Autodesk Fusion 360 part; units mm, degrees
note: some values were not read from the file. Chosen so that the rebuilt part matches the saved one: which face or edge a step refers to; the layout of a text. Set by a fixed rule: which sketch regions a step uses.
(part 2 of 2)
sketch "Sketch18" plane through (0, 0, -22.6) normal (0, 0, -1) x (1, 0, 0)
  line L0 (90.44, 31.25) -> (0.75, 31.25)
  arc A0 (0.75, 31.25) -> (-2.25, 28.25) centre (0.75, 28.25) ccw
  line L1 (-2.25, 28.25) -> (-2.25, 0.75)
  arc A1 (-2.25, 0.75) -> (0.75, -2.25) centre (0.75, 0.75) ccw
  line L2 (0.75, -2.25) -> (90.44, -2.25)
  arc A2 (90.44, -2.25) -> (93.44, 0.75) centre (90.44, 0.75) ccw
  line L3 (93.44, 0.75) -> (93.44, 28.25)
  arc A3 (93.44, 28.25) -> (90.44, 31.25) centre (90.44, 28.25) ccw
  line L4 (2.5, 13.75) -> (2.5, 12)
  line L5 (2.5, 12) -> (1, 12)
  line L6 (1, 12) -> (1, 13.75)
  line L7 (1, 13.75) -> (-0.75, 13.75)
  line L8 (-0.75, 13.75) -> (-0.75, 15.25)
  line L9 (-0.75, 15.25) -> (1, 15.25)
  line L10 (1, 15.25) -> (1, 17)
  line L11 (1, 17) -> (2.5, 17)
  line L12 (2.5, 17) -> (2.5, 15.25)
  line L13 (2.5, 15.25) -> (4.25, 15.25)
  line L14 (4.25, 15.25) -> (4.25, 13.75)
  line L15 (4.25, 13.75) -> (2.5, 13.75)
  line L16 (73.4403, 28.8585) -> (73.4403, 26.25)
  line L17 (73.4403, 26.25) -> (72.69, 26.25)
  line L18 (72.69, 26.25) -> (72.69, 30.25)
  line L19 (72.69, 30.25) -> (73.4758, 30.25)
  line L20 (73.4758, 30.25) -> (75.1129, 27.5788)
  line L21 (75.1129, 27.5788) -> (75.1129, 30.25)
  line L22 (75.1129, 30.25) -> (75.8633, 30.25)
  line L23 (75.8633, 30.25) -> (75.8633, 26.25)
  line L24 (75.8633, 26.25) -> (75.0529, 26.25)
  line L25 (75.0529, 26.25) -> (73.4403, 28.8585)
  spline S0 degree 3 poles (57.8412, 26.1791) (57.611, 26.1873) (57.1901, 26.2024) (56.8364, 26.4276) (56.6761, 26.5297) knots 0 0 0 0 0.067624 0.123634 0.123634 0.123634 0.123634
  spline S1 degree 3 poles (56.6761, 26.5297) (56.5536, 26.6663) (56.292, 26.958) (56.2257, 27.3455) (56.1905, 27.5515) knots 0 0 0 0 0.053943 0.115202 0.115202 0.115202 0.115202
  line L26 (56.1905, 27.5515) -> (56.9763, 27.6279)
  spline S2 degree 3 poles (56.9763, 27.6279) (57.0021, 27.5084) (57.0494, 27.2896) (57.1971, 27.1225) (57.2641, 27.0467) knots 0 0 0 0 0.035954 0.065825 0.065825 0.065825 0.065825
  spline S3 degree 3 poles (57.2641, 27.0467) (57.3465, 26.9927) (57.5236, 26.8765) (57.7359, 26.8665) (57.8494, 26.8612) knots 0 0 0 0 0.02903 0.062403 0.062403 0.062403 0.062403
  spline S4 degree 3 poles (57.8494, 26.8612) (57.9666, 26.8644) (58.1775, 26.8702) (58.3575, 26.9783) (58.4374, 27.0263) knots 0 0 0 0 0.034457 0.061988 0.061988 0.061988 0.061988
  spline S5 degree 3 poles (58.4374, 27.0263) (58.4951, 27.0818) (58.6055, 27.1883) (58.6256, 27.3399) (58.6352, 27.4123) knots 0 0 0 0 0.023254 0.044539 0.044539 0.044539 0.044539
  spline S6 degree 3 poles (58.6352, 27.4123) (58.6321, 27.4575) (58.626, 27.5455) (58.5763, 27.6183) (58.552, 27.6538) knots 0 0 0 0 0.013295 0.025956 0.025956 0.025956 0.025956
  spline S7 degree 3 poles (58.552, 27.6538) (58.5154, 27.6872) (58.4305, 27.7643) (58.3227, 27.8044) (58.2614, 27.8271) knots 0 0 0 0 0.014739 0.034108 0.034108 0.034108 0.034108
  spline S8 degree 3 poles (58.2614, 27.8271) (58.184, 27.8503) (57.9701, 27.9144) (57.7532, 27.9677) (57.6148, 28.0017) knots 0 0 0 0 0.02424 0.066991 0.066991 0.066991 0.066991
  spline S9 degree 3 poles (57.6148, 28.0017) (57.4253, 28.0498) (57.0991, 28.1327) (56.8203, 28.3192) (56.7034, 28.3973) knots 0 0 0 0 0.058092 0.099984 0.099984 0.099984 0.099984
  spline S10 degree 3 poles (56.7034, 28.3973) (56.596, 28.5125) (56.3836, 28.7401) (56.3511, 29.0494) (56.3351, 29.2023) knots 0 0 0 0 0.04588 0.090697 0.090697 0.090697 0.090697
  spline S11 degree 3 poles (56.3351, 29.2023) (56.3426, 29.3029) (56.3578, 29.5063) (56.4578, 29.6841) (56.5083, 29.7739) knots 0 0 0 0 0.029886 0.060385 0.060385 0.060385 0.060385
  spline S12 degree 3 poles (56.5083, 29.7739) (56.574, 29.8579) (56.7092, 30.031) (56.9063, 30.1288) (57.0077, 30.1791) knots 0 0 0 0 0.031562 0.065038 0.065038 0.065038 0.065038
  spline S13 degree 3 poles (57.0077, 30.1791) (57.1265, 30.2196) (57.3815, 30.3065) (57.651, 30.3141) (57.7948, 30.3182) knots 0 0 0 0 0.037465 0.080342 0.080342 0.080342 0.080342
  spline S14 degree 3 poles (57.7948, 30.3182) (58.0213, 30.3115) (58.4299, 30.2995) (58.7748, 30.0841) (58.9285, 29.9881) knots 0 0 0 0 0.06651 0.119965 0.119965 0.119965 0.119965
  spline S15 degree 3 poles (58.9285, 29.9881) (59.0404, 29.8666) (59.27, 29.6172) (59.3085, 29.2798) (59.3283, 29.1068) knots 0 0 0 0 0.048247 0.099032 0.099032 0.099032 0.099032
  line L27 (59.3283, 29.1068) -> (58.5206, 29.0713)
  spline S16 degree 3 poles (58.5206, 29.0713) (58.5017, 29.164) (58.4673, 29.3326) (58.3508, 29.4581) (58.2982, 29.5147) knots 0 0 0 0 0.027726 0.050455 0.050455 0.050455 0.050455
  spline S17 degree 3 poles (58.2982, 29.5147) (58.2288, 29.5539) (58.0708, 29.6431) (57.8887, 29.6474) (57.7867, 29.6497) knots 0 0 0 0 0.023601 0.053634 0.053634 0.053634 0.053634
  spline S18 degree 3 poles (57.7867, 29.6497) (57.6796, 29.6464) (57.4842, 29.6402) (57.313, 29.5472) (57.2355, 29.5051) knots 0 0 0 0 0.031585 0.057684 0.057684 0.057684 0.057684
  spline S19 degree 3 poles (57.2355, 29.5051) (57.1981, 29.4717) (57.1237, 29.4053) (57.1127, 29.3061) (57.1073, 29.2568) knots 0 0 0 0 0.014496 0.028843 0.028843 0.028843 0.028843
  spline S20 degree 3 poles (57.1073, 29.2568) (57.1128, 29.2108) (57.1243, 29.1159) (57.1923, 29.0486) (57.2273, 29.014) knots 0 0 0 0 0.013503 0.02781 0.02781 0.02781 0.02781
  spline S21 degree 3 poles (57.2273, 29.014) (57.3134, 28.9672) (57.5463, 28.8406) (57.8059, 28.7829) (57.9695, 28.7466) knots 0 0 0 0 0.029285 0.079208 0.079208 0.079208 0.079208
  spline S22 degree 3 poles (57.9695, 28.7466) (58.1423, 28.7051) (58.4411, 28.6334) (58.7225, 28.5105) (58.8412, 28.4587) knots 0 0 0 0 0.05318 0.09196 0.09196 0.09196 0.09196
  spline S23 degree 3 poles (58.8412, 28.4587) (58.9299, 28.4052) (59.1048, 28.2996) (59.2243, 28.1339) (59.2832, 28.0522) knots 0 0 0 0 0.030713 0.060609 0.060609 0.060609 0.060609
  spline S24 degree 3 poles (59.2832, 28.0522) (59.3298, 27.9578) (59.4286, 27.7573) (59.4379, 27.5335) (59.4429, 27.4151) knots 0 0 0 0 0.031207 0.066326 0.066326 0.066326 0.066326
  spline S25 degree 3 poles (59.4429, 27.4151) (59.4346, 27.3019) (59.418, 27.0733) (59.3076, 26.8725) (59.2519, 26.7711) knots 0 0 0 0 0.033629 0.067874 0.067874 0.067874 0.067874
  spline S26 degree 3 poles (59.2519, 26.7711) (59.1807, 26.6771) (59.0359, 26.4859) (58.8209, 26.3793) (58.7116, 26.325) knots 0 0 0 0 0.03487 0.070919 0.070919 0.070919 0.070919
  spline S27 degree 3 poles (58.7116, 26.325) (58.5819, 26.2825) (58.2995, 26.19) (58.0021, 26.1829) (57.8412, 26.1791) knots 0 0 0 0 0.040722 0.088678 0.088678 0.088678 0.088678
  line L28 (90.065, 17) -> (90.065, 12)
  line L29 (90.065, 12) -> (88.565, 12)
  line L30 (88.565, 12) -> (88.565, 17)
  line L31 (88.565, 17) -> (90.065, 17)
  arc A4 (59.69, 25) -> (61.19, 26.5) centre (59.69, 26.5) ccw
  line L32 (61.19, 26.5) -> (61.19, 28.5)
  arc A5 (62.69, 30) -> (61.19, 28.5) centre (62.69, 28.5) ccw
  line L33 (62.69, 30) -> (70.19, 30)
  arc A6 (71.69, 28.5) -> (70.19, 30) centre (70.19, 28.5) ccw
  line L34 (71.69, 28.5) -> (71.69, 27.5)
  line L35 (73.19, 26) -> (83.69, 26)
  line L36 (85.19, 24.5) -> (85.19, 4.5)
  arc A7 (83.69, 3) -> (85.19, 4.5) centre (83.69, 4.5) ccw
  line L37 (83.69, 3) -> (7.5, 3)
  arc A8 (6, 4.5) -> (7.5, 3) centre (7.5, 4.5) ccw
  line L38 (6, 4.5) -> (6, 23.5)
  arc A9 (7.5, 25) -> (6, 23.5) centre (7.5, 23.5) ccw
  line L39 (7.5, 25) -> (59.69, 25)
  circle A10 centre (1.97, 2) radius 3 construction
  circle A11 centre (89.22, 2) radius 3 construction
  circle A12 centre (89.22, 27) radius 3 construction
  circle A13 centre (1.97, 27) radius 3 construction
  circle A14 centre (89.22, 2) radius 2.6
  circle A15 centre (1.97, 2) radius 2.6
  circle A16 centre (1.97, 27) radius 2.6
  circle A17 centre (89.22, 27) radius 2.6
  arc A18 (6.1, 4.5) -> (7.5, 3.1) centre (7.5, 4.5) ccw
  line L40 (83.69, 3.1) -> (7.5, 3.1)
  arc A19 (83.69, 3.1) -> (85.09, 4.5) centre (83.69, 4.5) ccw
  line L41 (85.09, 23.5) -> (85.09, 4.5)
  arc A20 (85.09, 23.5) -> (83.69, 24.9) centre (83.69, 23.5) ccw
  line L42 (73.19, 24.9) -> (83.69, 24.9)
  arc A21 (71.59, 26.5) -> (73.19, 24.9) centre (73.19, 26.5) ccw
  line L43 (71.59, 28.5) -> (71.59, 26.5)
  arc A22 (71.59, 28.5) -> (70.19, 29.9) centre (70.19, 28.5) ccw
  line L44 (62.69, 29.9) -> (70.19, 29.9)
  arc A23 (62.69, 29.9) -> (61.29, 28.5) centre (62.69, 28.5) ccw
  line L45 (61.29, 26.5) -> (61.29, 28.5)
  arc A24 (59.69, 24.9) -> (61.29, 26.5) centre (59.69, 26.5) ccw
  line L46 (7.5, 24.9) -> (59.69, 24.9)
  arc A25 (7.5, 24.9) -> (6.1, 23.5) centre (7.5, 23.5) ccw
  line L47 (6.1, 4.5) -> (6.1, 23.5)
  line L48 (5.5, 31.25) -> (0.75, 31.25)
  arc A26 (0.75, 31.25) -> (-2.25, 28.25) centre (0.75, 28.25) ccw
  line L49 (-2.25, 28.25) -> (-2.25, 0.75)
  arc A27 (-2.25, 0.75) -> (0.75, -2.25) centre (0.75, 0.75) ccw
  line L50 (0.75, -2.25) -> (6.5, -2.25)
  line L51 (15.5, -2.25) -> (90.44, -2.25)
  line L52 (15.5, -2.25) -> (6.5, -2.25)
  arc A28 (90.44, -2.25) -> (93.44, 0.75) centre (90.44, 0.75) ccw
  line L53 (93.44, 0.75) -> (93.44, 28.25)
  arc A29 (93.44, 28.25) -> (90.44, 31.25) centre (90.44, 28.25) ccw
  line L54 (90.44, 31.25) -> (15.5, 31.25)
  line L55 (5.5, 31.25) -> (15.5, 31.25)
  line L56 (59.69, 24.9) -> (73.19, 24.9)
  arc A30 (71.69, 27.5) -> (73.19, 26) centre (73.19, 27.5) ccw
  arc A31 (85.19, 24.5) -> (83.69, 26) centre (83.69, 24.5) ccw
  dimension "d144" = 5.2
  constraint concentric A11 A14
  constraint concentric A10 A15
  constraint concentric A13 A16
  constraint concentric A12 A17
  constraint equal A14 A15
  constraint equal A15 A16
  constraint equal A16 A17
  constraint concentric A8 A18
  constraint parallel L37 L40
  constraint concentric A7 A19
  constraint parallel L36 L41
  constraint parallel L35 L42
  constraint parallel L34 L43
  constraint concentric A6 A22
  constraint parallel L33 L44
  constraint concentric A5 A23
  constraint parallel L32 L45
  constraint concentric A4 A24
  constraint parallel L39 L46
  constraint concentric A9 A25
  constraint parallel L38 L47
  constraint tangent A18 L47
  constraint tangent A18 L40
  constraint tangent L42 A21
  constraint tangent L40 A19
  constraint tangent A19 L41
  constraint tangent L41 A20
  constraint tangent A20 L42
  constraint tangent A21 L43
  constraint tangent L43 A22
  constraint tangent A22 L44
  constraint tangent L44 A23
  constraint tangent A23 L45
  constraint tangent L45 A24
  constraint tangent A24 L46
  constraint tangent L46 A25
  constraint tangent A25 L47
  measures "d144" diameter of A14
extrude "Extrude21" cut sketch "Sketch18" against normal blind 2.7 contours A14 | A15 | A16 | A17 bodies 2
extrude "Extrude22" add sketch "Sketch18" along normal blind 2.7 separate body contours L0 A0 L1 A1 L2 A2 L3 A3 L48 A26 L49 A27 L50 L51 L52 A28 L53 A29 L54 L55 | L4 L5 L6 L7 L8 L9 L10 L11 L12 L13 L14 L15 | L16 L17 L18 L19 L20 L21 L22 L23 L24 L25 | S0 S1 L26 S2 S3 S4 S5 S6 S7 S8 S9 S10 S11 S12 S13 S14 S15 L27 S16 S17 S18 S19 S20 S21 S22 S23 S24 S25 S26 S27 | L28 L29 L30 L31 | A4 L32 A5 L33 A6 L34 L35 L36 A7 L37 A8 L38 A9 L39 A30 A31 | A18 L40 A19 L41 A20 L42 L46 A25 L47 L56 | A21 L43 A22 L44 A23 L45 A24 L56 makes body 3
extrude "Extrude23" add sketch "Sketch18" along normal blind 1 from surface at 2.7 contours L0 A0 L1 A1 L2 A2 L3 A3 L48 A26 L49 A27 L50 L51 L52 A28 L53 A29 L54 L55 | L4 L5 L6 L7 L8 L9 L10 L11 L12 L13 L14 L15 | L16 L17 L18 L19 L20 L21 L22 L23 L24 L25 | S0 S1 L26 S2 S3 S4 S5 S6 S7 S8 S9 S10 S11 S12 S13 S14 S15 L27 S16 S17 S18 S19 S20 S21 S22 S23 S24 S25 S26 S27 | L28 L29 L30 L31 | A4 L32 A5 L33 A6 L34 L35 L36 A7 L37 A8 L38 A9 L39 A30 A31 | A14 | A15 | A16 | A17 | A18 L40 A19 L41 A20 L42 L46 A25 L47 L56 | A21 L43 A22 L44 A23 L45 A24 L56 bodies 3
extrude "Extrude24" add sketch "Sketch18" against normal blind 0.5 contours A18 L40 A19 L41 A20 L42 L46 A25 L47 L56 bodies 3
fillet "Fillet8" radius 1 8 edges at (84.69, 0.5, 1.7) (84.69, -3.5, 2.5) (79.69, -3.5, 2.5) (79.69, 0.5, 1.7) (79.69, -23.5, 2.5) (84.69, -23.5, 2.5) (84.69, -27.5, 2.5) (79.69, -27.5, 2.5) on bodies 1
sketch "Sketch19" plane through (0, 2.25, 0) normal (0, 1, 0) x (-1, 0, 0)
  line L0 (-0.75, -1.6) -> (-90.44, -1.6)
  line L1 (-90.44, -1.6) -> (-90.44, -22.6)
  line L2 (-90.44, -22.6) -> (-0.75, -22.6)
  line L3 (-0.75, -22.6) -> (-0.75, -1.6)
  line L4 (-90.44, -22.6) -> (-0.75, -22.6) construction
  line L5 (-0.75, -22.6) -> (-0.75, -1.6) construction
  line L6 (-0.75, -1.6) -> (-90.44, -1.6) construction
  line L7 (-90.44, -1.6) -> (-90.44, -22.6) construction
  text T0 "TASMOTA" font "Arial" height 10 bold align centre middle in box 89.69 x 21 at (-90.44, -22.6) x (1, 0) y (0, 1) spacing 1 kerned
  constraint midpoint L1
  constraint midpoint L3 L5
  constraint midpoint L0 L6
extrude "Extrude25" cut sketch "Sketch19" against normal blind 0.2 text T0 bodies 2
sketch "Sketch20" plane through (0, -31.25, 0) normal (0, -1, 0) x (1, 0, 0)
  line L0 (90.44, -1.6) -> (0.75, -1.6)
  line L1 (0.75, -1.6) -> (0.75, -22.6)
  line L2 (0.75, -22.6) -> (90.44, -22.6)
  line L3 (90.44, -22.6) -> (90.44, -1.6)
  line L4 (0.75, -22.6) -> (90.44, -22.6) construction
  line L5 (90.44, -22.6) -> (90.44, -1.6) construction
  line L6 (90.44, -1.6) -> (0.75, -1.6) construction
  line L7 (0.75, -1.6) -> (0.75, -22.6) construction
  text T0 "BME280" font "Arial" height 10 bold align centre middle in box 89.69 x 21 at (0.75, -22.6) x (1, 0) y (0, 1) spacing 1
  constraint coincident L2
  constraint midpoint L1
  constraint midpoint L0 L6
extrude "Extrude26" cut sketch "Sketch20" against normal blind 0.2 text T0 bodies 2
equation "d4 = 90.25 mm - 6 mm"
equation "d5 = 28 mm - 6 mm"
equation "d123 = 1 mm - 0.317 mm"
named bodies: "T-Energy Thicc Top", "T-Energy Thicc Middle", "T-Energy Thicc Bottom"
